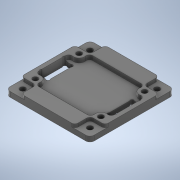
# Autodesk Inventor part: Camera_root_frame_KBCR-S02MU
Saved by Autodesk Inventor 2020.4 (Build 244396000, 396)
## iProperties
Part Number: Camera_root_frame_KBCR-S02MU
Material: アセタール樹脂、黒
Document SubType Name: Modeling
Designer: Masato Kubotera
Density: 1.425 g/cm^3
Appearance: 滑らか - 黒
Description: POM T5
Mass: 8.58066 g
Surface Area: 62.5532 cm^2
Volume: 6.02152 cm^3
Author: Masato Kubotera
Autodesk Inventor part; units mm, degrees
ref_plane "YZ Plane" through (0, 0, 0) normal (1, 0, 0) x (0, 1, 0)
ref_plane "XZ Plane" through (0, 0, 0) normal (0, 1, 0) x (-1, 0, 0)
ref_plane "XY Plane" through (0, 0, 0) normal (0, 0, 1) x (1, 0, 0)
derived "KBCR-S02MU.ipt"
sketch "スケッチ2" plane through (0, 0, 0) normal (0, 0, 1) x (1, 0, 0)
  line L0 (-22.5, 25) -> (22.5, 25)
  line L1 (25, 22.5) -> (25, -22.5)
  line L2 (22.5, -25) -> (-22.5, -25)
  line L3 (-25, -22.5) -> (-25, 22.5)
  line L4 (-25, 25) -> (25, -25) construction
  line L5 (25, 25) -> (-25, -25) construction
  arc A0 (-22.5, 25) -> (-25, 22.5) centre (-22.5, 22.5) ccw
  arc A1 (-25, -22.5) -> (-22.5, -25) centre (-22.5, -22.5) ccw
  arc A2 (22.5, -25) -> (25, -22.5) centre (22.5, -22.5) ccw
  arc A3 (25, 22.5) -> (22.5, 25) centre (22.5, 22.5) ccw
  line L6 (-25, -22.5) -> (25, -22.5) construction
  line L7 (25, -22.5) -> (25, -17.5)
  line L8 (25, -17.5) -> (-25, -17.5) construction
  line L9 (-25, -17.5) -> (-25, -22.5) construction
  line L10 (-25, -22.5) -> (25, -17.5) construction
  line L11 (25, -22.5) -> (-25, -17.5) construction
  line L12 (-25, -20) -> (25, -20) construction
  line L13 (0, 22.5) -> (0, -22.5) construction
  circle A4 centre (-20, -20) radius 1.6
  circle A5 centre (20, -20) radius 1.6
  line L14 (-16, 0) -> (16, 0) construction
  circle A6 centre (-20, 20) radius 1.6
  circle A7 centre (20, 20) radius 1.6
  circle A8 centre (-5.5, -9) radius 2 construction
  circle A9 centre (13, 19.5) radius 1.1 projected
  circle A10 centre (13, -19.5) radius 1.1 projected
  circle A11 centre (-13, -19.5) radius 1.1 projected
  circle A12 centre (-13, 19.5) radius 1.1 projected
  circle A13 centre (-13, -19.5) radius 1.55
  circle A14 centre (13, -19.5) radius 1.55
  circle A15 centre (13, 19.5) radius 1.55
  circle A16 centre (-13, 19.5) radius 1.55
  line L15 (-14, -22.5) -> (14, -22.5) projected
  line L16 (-16, 20.5) -> (-16, -20.5) projected
  line L17 (-16, -14.3461) -> (-16, 0)
  line L18 (0, -22.5) -> (-7.8461, -22.5)
  arc A17 (-9.8095, -20.119) -> (-13.619, -16.3095) centre (-13, -19.5) ccw
  arc A18 (-9.8095, -20.119) -> (-7.8461, -22.5) centre (-7.8461, -20.5) ccw
  arc A19 (-16, -14.3461) -> (-13.619, -16.3095) centre (-14, -14.3461) ccw
  line L19 (-16, 14.3461) -> (-16, 0)
  line L20 (0, 22.5) -> (-7.8461, 22.5)
  arc A20 (-13.619, 16.3095) -> (-9.8095, 20.119) centre (-13, 19.5) ccw
  arc A21 (-7.8461, 22.5) -> (-9.8095, 20.119) centre (-7.8461, 20.5) ccw
  arc A22 (-13.619, 16.3095) -> (-16, 14.3461) centre (-14, 14.3461) ccw
  line L21 (16, -14.3461) -> (16, 0)
  line L22 (0, -22.5) -> (7.8461, -22.5)
  arc A23 (13.619, -16.3095) -> (9.8095, -20.119) centre (13, -19.5) ccw
  arc A24 (7.8461, -22.5) -> (9.8095, -20.119) centre (7.8461, -20.5) ccw
  arc A25 (13.619, -16.3095) -> (16, -14.3461) centre (14, -14.3461) ccw
  arc A26 (16, 14.3461) -> (13.619, 16.3095) centre (14, 14.3461) ccw
  arc A27 (9.8095, 20.119) -> (7.8461, 22.5) centre (7.8461, 20.5) ccw
  line L23 (16, 14.3461) -> (16, 0)
  line L24 (0, 22.5) -> (7.8461, 22.5)
  arc A28 (9.8095, 20.119) -> (13.619, 16.3095) centre (13, 19.5) ccw
  line L25 (-7.5, -22.5) -> (7.5, -22.5) construction
  line L26 (7.5, -22.5) -> (7.5, -17.5) construction
  line L27 (7.5, -17.5) -> (-7.5, -17.5) construction
  line L28 (-7.5, -17.5) -> (-7.5, -22.5) construction
  line L29 (-7.5, -22.5) -> (7.5, -17.5) construction
  line L30 (7.5, -22.5) -> (-7.5, -17.5) construction
  line L31 (-6.0651, -22.55) -> (6.0651, -22.55)
  line L32 (6.0651, -17.45) -> (-6.0651, -17.45)
  arc A29 (-7.55, -21.0651) -> (-6.0651, -22.55) centre (-6.8075, -21.8075) ccw
  arc A30 (-6.0651, -17.45) -> (-7.55, -18.9349) centre (-6.8075, -18.1925) ccw
  arc A31 (6.0651, -22.55) -> (7.55, -21.0651) centre (6.8075, -21.8075) ccw
  arc A32 (7.55, -18.9349) -> (6.0651, -17.45) centre (6.8075, -18.1925) ccw
  line L33 (-7.55, -22.5) -> (-7.55, -22.55)
  line L34 (-7.55, -18.9349) -> (-7.55, -21.0651)
  line L35 (7.55, -21.0651) -> (7.55, -18.9349)
  line L36 (-6.0651, 22.55) -> (6.0651, 22.55)
  line L37 (6.0651, 17.45) -> (-6.0651, 17.45)
  arc A33 (-6.0651, 22.55) -> (-7.55, 21.0651) centre (-6.8075, 21.8075) ccw
  arc A34 (-7.55, 18.9349) -> (-6.0651, 17.45) centre (-6.8075, 18.1925) ccw
  arc A35 (6.0651, 17.45) -> (7.55, 18.9349) centre (6.8075, 18.1925) ccw
  arc A36 (7.55, 21.0651) -> (6.0651, 22.55) centre (6.8075, 21.8075) ccw
  line L38 (-7.55, 18.9349) -> (-7.55, 21.0651)
  line L39 (7.55, 21.0651) -> (7.55, 18.9349)
  arc A37 (-16, -18) -> (-18, -16) centre (-18, -18) ccw
  line L40 (-16, -18) -> (-16, -23)
  arc A38 (-15.9998, -22.9729) -> (-14, -25) centre (-14, -23) ccw
  line L41 (-16, 18) -> (-16, 23)
  arc A39 (-14, 25) -> (-15.9998, 22.9729) centre (-14, 23) ccw
  line L42 (16, -18) -> (16, -23)
  arc A40 (14, -25) -> (15.9998, -22.9729) centre (14, -23) ccw
  line L43 (16, 18) -> (16, 23)
  arc A41 (15.9998, 22.9729) -> (14, 25) centre (14, 23) ccw
  line L44 (-16, 14.3461) -> (-16, -14.3461)
  line L45 (16, 14.3461) -> (16, -14.3461)
  line L46 (16, 0) -> (-16, 0) construction
  arc A42 (-25, -14) -> (-23, -16) centre (-23, -14) ccw
  line L47 (-23, -16) -> (-18, -16)
  arc A43 (-18, 16) -> (-16, 18) centre (-18, 18) ccw
  arc A44 (-23, 16) -> (-25, 14) centre (-23, 14) ccw
  line L48 (-23, 16) -> (-18, 16)
  arc A45 (18, -16) -> (16, -18) centre (18, -18) ccw
  arc A46 (23, -16) -> (25, -14) centre (23, -14) ccw
  line L49 (23, -16) -> (18, -16)
  arc A47 (25, 14) -> (23, 16) centre (23, 14) ccw
  line L50 (23, 16) -> (18, 16)
  arc A48 (16, 18) -> (18, 16) centre (18, 18) ccw
  point P0 (0, 0)
  point P1 (0, -20)
  point P2 (0, -20)
  point P3 (-11.75, -22.5)
  point P4 (-16, -14.3461)
  point P5 (-16, 14.3461)
  point P6 (7.8461, -22.5)
  point P7 (-7.8461, -22.5)
  point P8 (-16.5858, -16.5858)
  point P9 (14, -25)
  point P10 (14, 25)
  point P11 (-14, 25)
  point P12 (-25, 14)
  point P13 (25, 14)
  point P14 (-7.5968, -22.5)
  point P15 (7.5968, -22.5)
  point P16 (7.5968, 22.5)
  point P17 (-7.5968, 22.5)
  dimension "d1" = 50
  dimension "d2" = 50
  dimension "d3" = 2.5
  dimension "d7" = 5
  dimension "d8" = 5
  dimension "d9" = 3.2
  dimension "d10" = 5
  dimension "d12" = 3.1
  dimension "d20" = 2
  dimension "d21" = 40
  dimension "d23" = 12.5
  dimension "d24" = 15
  dimension "d27" = 0.05
  dimension "d28" = 1.05
  dimension "d30" = 0.05
  dimension "d33" = 9
  dimension "d39" = 2
  dimension "d40" = 2
  dimension "d41" = 4
  dimension "d46" = 16
  dimension "d59" = 4
  dimension "d60" = 2
  dimension "d61" = 3.25
  constraints: 94 end point, 79 point on circle, 79 symmetric about line, 44 centre point, 21 point on line, 18 tangent, 10 parallel, 9 midpoint, 5 coincident, 4 equal radius, 4 horizontal, 4 perpendicular, 2 collinear, 1 vertical, 31 other
  measures "d1" distance of L4.end L5.end
  measures "d2" distance of L5.start L4.end
  measures "d3" radius of A0
  measures "d7" distance of L7.end L6.end
  measures "d8" distance from line of L5.end L12
  measures "d9" diameter of A4
  measures "d10" distance of L12.start A4.centre
  measures "d12" diameter of A13
  measures "d20" radius of A18
  measures "d21" distance of A6.centre A4.centre
  measures "d23" horizontal distance of L25.start A4.centre
  measures "d24" distance of L25.end L25.start
  measures "d27" distance between parallel lines of L31 L25
  measures "d28" radius of A29
  measures "d30" distance between parallel lines of L28 L34
  measures "d33" distance from line of L1 L14.end
  measures "d39" radius of A38
  measures "d40" radius of A37
  measures "d41" horizontal distance of L40.end A4.centre
  measures "d46" distance of point (0, 0) L14.start
  measures "d59" distance from line of A4.centre L47
  measures "d60" radius of A42
  measures "d61" radius of A17
extrude "押し出し1" add sketch "スケッチ2" along normal blind 5 contours L0 A41 L43 A48 L50 A47 L1 A46 L49 A45 L42 A40 L2 A38 L40 L16 A19 A17 A18 L15 A29 L31 A31 A24 A23 A25 L21 L23 A26 A28 A27 L24 A36 L36 A33 L20 A21 A20 A22 L41 A39 | A44 L48 A43 L16 A37 L47 A42 L3
extrude "押し出し2" add sketch "スケッチ2" along normal blind 2.5 contours A22 A20 A21 L20 A33 L38 A34 L37 A35 L39 A36 L24 A27 A28 A26 L23 L21 A25 A23 A24 L15 A31 L35 A32 L32 A30 L34 A29 A18 A17 A19 L16
extrude "押し出し3" add sketch "スケッチ2" along normal blind 3 contours L0 A39 L41 L16 A43 L48 A44 L3 A0 | L0 A3 L1 A47 L50 A48 L43 A41 | A42 L47 A37 L16 L40 A38 L2 A1 L3 | L1 A2 L2 A40 L42 A45 L49 A46
sketch "スケッチ1" plane through (0, 0, 0) normal (0, 0, 1) x (1, 0, 0)
  line L0 (14, 22.5) -> (-14, 22.5) construction
  line L1 (-16, 20.5) -> (-16, -20.5) construction
  line L2 (-14, -22.5) -> (14, -22.5) construction
  line L3 (16, -20.5) -> (16, 20.5) construction
  line L4 (16, 22.5) -> (-16, -22.5) construction
  line L5 (-16, 22.5) -> (16, -22.5) construction
  line L6 (-13, 19.5) -> (13, 19.5) construction
  line L7 (13, 19.5) -> (13, -19.5) construction
  line L8 (13, -19.5) -> (-13, -19.5) construction
  line L9 (-13, -19.5) -> (-13, 19.5) construction
  line L10 (-13, 19.5) -> (13, -19.5) construction
  line L11 (13, 19.5) -> (-13, -19.5) construction
  circle A0 centre (-13, -19.5) radius 1.1 construction
  line L12 (-16, 0) -> (16, 0) construction
  line L13 (0, 22.5) -> (0, -22.5) construction
  circle A1 centre (-13, 19.5) radius 1.1 construction
  circle A2 centre (13, 19.5) radius 1.1 construction
  circle A3 centre (13, -19.5) radius 1.1 construction
  circle A4 centre (-13, -19.5) radius 2 construction
  circle A5 centre (-13, 19.5) radius 2 construction
  circle A6 centre (13, -19.5) radius 2 construction
  circle A7 centre (13, 19.5) radius 2 construction
  circle A8 centre (0, 0) radius 7.25 construction
  circle A9 centre (-5.5, -9) radius 2 construction
  arc A10 (-16, -20.5) -> (-14, -22.5) centre (-14, -20.5) ccw construction
  arc A11 (14, -22.5) -> (16, -20.5) centre (14, -20.5) ccw construction
  arc A12 (16, 20.5) -> (14, 22.5) centre (14, 20.5) ccw construction
  arc A13 (-14, 22.5) -> (-16, 20.5) centre (-14, 20.5) ccw construction
  line L14 (-10.5, 11.5) -> (10.5, 11.5) projected
  line L15 (11.5, 10.5) -> (11.5, -10.5) projected
  line L16 (10.5, -11.5) -> (-10.5, -11.5) projected
  line L17 (-11.5, -10.5) -> (-11.5, 10.5) projected
  line L18 (-11.5, 11.5) -> (11.5, -11.5) construction
  line L19 (11.5, 11.5) -> (-11.5, -11.5) construction
  line L20 (3.85, -24.5) -> (-3.85, -24.5) projected
  line L21 (-3.85, -24.5) -> (-3.85, -15.5) projected
  line L22 (-3.85, -15.5) -> (3.85, -15.5) projected
  line L23 (3.85, -15.5) -> (3.85, -24.5) projected
  line L24 (3.85, -24.5) -> (-3.85, -15.5) construction
  line L25 (-3.85, -24.5) -> (3.85, -15.5) construction
  line L26 (-4.5, 21.5) -> (4.5, 21.5) projected
  line L27 (4.5, 21.5) -> (4.5, 15) projected
  line L28 (4.5, 15) -> (-4.5, 15) projected
  line L29 (-4.5, 15) -> (-4.5, 21.5) projected
  line L30 (-4.5, 21.5) -> (4.5, 15) construction
  line L31 (4.5, 21.5) -> (-4.5, 15) construction
  arc A14 (-10.5, 11.5) -> (-11.5, 10.5) centre (-10.5, 10.5) ccw projected
  arc A15 (-11.5, -10.5) -> (-10.5, -11.5) centre (-10.5, -10.5) ccw projected
  arc A16 (10.5, -11.5) -> (11.5, -10.5) centre (10.5, -10.5) ccw projected
  arc A17 (11.5, 10.5) -> (10.5, 11.5) centre (10.5, 10.5) ccw projected
  arc A18 (-12.5, 2) -> (-12.5, -2) centre (-12.5, 0) ccw projected
  line L32 (-12.5, 2) -> (-11.5, 2) projected
  line L33 (-12.5, -2) -> (-11.5, -2) projected
  line L34 (12.5, 2) -> (11.5, 2) projected
  arc A19 (12.5, -2) -> (12.5, 2) centre (12.5, 0) ccw projected
  line L35 (12.5, -2) -> (11.5, -2) projected
  point P0 (0, -20)
  point P1 (0, 18.25)
  constraints: 1 centre point
equation "\"d27\" = d26"
equation "\"d40\" = d39"
equation "\"d26\" = 0.05"
